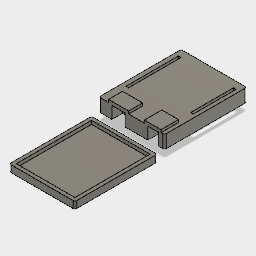
TentativeArduinoCase (Autodesk Fusion 360 design; units mm, degrees)
Autodesk Fusion 360 part; units mm, degrees
sketch "Sketch1" plane through (0, 0, 0) normal (0, 1, 0) x (1, 0, 0)
  line L0 (0, 0) -> (59.5312, 0)
  line L1 (59.5312, 0) -> (59.5312, 74.6125)
  line L2 (59.5312, 74.6125) -> (0, 74.6125)
  line L3 (0, 74.6125) -> (0, 0)
  dimension "d1" = 59.5312
  dimension "d2" = 74.6125
  constraint horizontal L0
  constraint vertical L1
  constraint horizontal L2
  constraint vertical L3
  constraint coincident L0.start L3.end
extrude "Extrude1" add sketch "Sketch1" against normal blind 6.35 makes body 1
sketch "Sketch2" plane through (0, 0, 0) normal (0, 1, 0) x (-1, 0, 0)
  line L0 (0, -74.6125) -> (0, 0)
  line L1 (0, 0) -> (-59.5312, 0)
  line L2 (-59.5312, 0) -> (-59.5312, -74.6125)
  line L3 (-59.5312, -74.6125) -> (0, -74.6125)
  line L4 (-56.3562, 0) -> (-41.275, 0)
  line L5 (-41.275, 0) -> (-56.3562, 0)
  line L6 (-41.275, 0) -> (-50.0063, 0)
  line L7 (-41.275, 0) -> (-56.3626, 0)
  line L8 (-56.3626, 0) -> (-56.3626, -15.875)
  line L9 (-56.3626, -15.875) -> (-41.275, -15.875)
  line L10 (-41.275, -15.875) -> (-41.275, 0)
  dimension "d6" = 15.0813
  dimension "d30" = 18.2563
  dimension "d31" = 15.875
  dimension "d93" = 15.0876
  constraint horizontal L6
  constraint horizontal L7
  constraint vertical L8
  constraint horizontal L9
  constraint vertical L10
  measures "d31" distance of L0.end
  measures "d93" distance of L8 L10
extrude "Extrude2" add sketch "Sketch2" along normal blind 14.2875 contours L1 L4 L5 L6 L7 L8 L9 L10 bodies 1
sketch "Sketch3" plane through (0, 0, 0) normal (0, 1, 0) x (-1, 0, 0)
  line L0 (-56.3626, 0) -> (-59.5312, 0)
  line L1 (-59.5312, 0) -> (-59.5312, -74.6125)
  line L2 (-59.5312, -74.6125) -> (0, -74.6125)
  line L3 (0, -74.6125) -> (0, 0)
  line L4 (0, 0) -> (-41.275, 0)
  line L5 (0, 0) -> (-26.9875, 0)
  line L6 (-26.9875, 0) -> (-8.7313, 0)
  line L7 (-8.7313, 0) -> (-20.6375, 0)
  line L8 (-8.7313, -12.7) -> (-8.7313, 0)
  line L9 (-56.3626, -15.875) -> (-56.3626, 0)
  line L10 (-41.275, 0) -> (-41.275, -15.875)
  line L11 (-41.275, -15.875) -> (-56.3626, -15.875)
  line L12 (-8.7313, -12.7) -> (-26.9875, -12.7)
  line L13 (-26.9875, -12.7) -> (-26.9875, 0)
  line L14 (-26.9875, 0) -> (-8.7313, 0)
  line L15 (-8.7313, 0) -> (-8.7313, -12.7)
  dimension "d10" = 26.9875
  dimension "d11" = 18.2563
  dimension "d12" = 12.7
  constraint coincident L3.end L4.start
  constraint coincident L5 L3.end
  constraint coincident L4 L3.end
  constraint horizontal L7
  constraint vertical L8
  constraint horizontal L12
  constraint vertical L13
  constraint horizontal L14
  constraint vertical L15
  measures "d12" distance of L3.end
extrude "Extrude3" add sketch "Sketch3" along normal blind 14.2875 contours L4 L5 L6 L7 L8 L12 L13 L14 L15 bodies 1
sketch "Sketch12" plane through (0, 0, 0) normal (0, 1, 0) x (-1, 0, 0)
  line L0 (-26.9875, -12.7) -> (-26.9875, 0)
  line L1 (-26.9875, 0) -> (-41.275, 0)
  line L2 (-41.275, 0) -> (-41.275, -15.875)
  line L3 (-41.275, -15.875) -> (-56.3626, -15.875)
  line L4 (-56.3626, -15.875) -> (-56.3626, 0)
  line L5 (-56.3626, 0) -> (-59.5312, 0)
  line L6 (-59.5312, 0) -> (-59.5312, -74.6125)
  line L7 (-59.5312, -74.6125) -> (0, -74.6125)
  line L8 (0, -74.6125) -> (0, 0)
  line L9 (0, 0) -> (-8.7313, 0)
  line L10 (-8.7313, 0) -> (-8.7313, -12.7)
  line L11 (-8.7313, -12.7) -> (-26.9875, -12.7)
  line L12 (0, 0) -> (-8.7313, 0)
  line L13 (-8.7313, 0) -> (-8.7313, -7.9375)
  line L14 (-8.7313, -7.9375) -> (0, -7.9375)
  line L15 (0, -7.9375) -> (0, 0)
  dimension "d57" = 7.9375
  constraint horizontal L12
  constraint vertical L13
  constraint horizontal L14
  constraint vertical L15
  constraint coincident L8.end L9.start
  measures "d57" distance of L8.end
extrude "Extrude10" add sketch "Sketch12" along normal blind 11.9062 bodies 1
sketch "Sketch13" plane through (0, 11.9062, 0) normal (0, 1, 0) x (-1, 0, 0)
  line L0 (-8.7313, -12.7) -> (-26.9875, -12.7)
  line L1 (-26.9875, -12.7) -> (-26.9875, 0)
  line L2 (0, 0) -> (-8.7313, 0)
  line L3 (-41.275, 0) -> (-41.275, -15.875)
  line L4 (-41.275, -15.875) -> (-56.3626, -15.875)
  line L5 (-56.3626, -15.875) -> (-56.3626, 0)
  line L6 (-56.3626, 0) -> (-59.5312, 0)
  line L7 (-59.5312, 0) -> (-59.5312, -74.6125)
  line L8 (-59.5312, -74.6125) -> (0, -74.6125)
  line L9 (0, -74.6125) -> (0, 0)
  line L10 (-8.7313, 0) -> (-8.7313, -12.7)
  line L11 (0, -74.6125) -> (-6.35, -74.6125)
  line L12 (-6.35, -74.6125) -> (-6.35, -20.6375)
  line L13 (-6.35, -20.6375) -> (0, -20.6375)
  line L14 (0, -20.6375) -> (0, -74.6125)
  line L15 (-59.5312, -74.6125) -> (-53.975, -74.6125)
  line L16 (-53.975, -74.6125) -> (-53.975, -29.3688)
  line L17 (-53.975, -29.3688) -> (-59.5312, -29.3688)
  line L18 (-59.5312, -29.3688) -> (-59.5312, -74.6125)
  line L19 (-26.9875, 0) -> (-41.275, 0)
  line L20 (0, -74.6125) -> (-3.9688, -74.6125)
  line L21 (-3.9688, -74.6125) -> (-3.9688, -20.6375)
  line L22 (-3.9688, -20.6375) -> (0, -20.6375)
  line L23 (0, -20.6375) -> (0, -74.6125)
  line L24 (0, -74.6125) -> (-6.35, -74.6125)
  line L25 (-6.35, -74.6125) -> (-6.35, -68.2625)
  line L26 (-6.35, -68.2625) -> (0, -68.2625)
  line L27 (0, -68.2625) -> (0, -74.6125)
  line L28 (-59.5312, -74.6125) -> (-56.3563, -74.6125)
  line L29 (-56.3563, -74.6125) -> (-56.3563, -29.3688)
  line L30 (-56.3563, -29.3688) -> (-59.5312, -29.3688)
  line L31 (-59.5312, -29.3688) -> (-59.5312, -74.6125)
  line L32 (-59.5312, -74.6125) -> (-53.975, -74.6125)
  line L33 (-53.975, -74.6125) -> (-53.975, -68.2625)
  line L34 (-53.975, -68.2625) -> (-59.5312, -68.2625)
  line L35 (-59.5312, -68.2625) -> (-59.5312, -74.6125)
  dimension "d60" = 53.975
  dimension "d61" = 6.35
  dimension "d62" = 45.2437
  dimension "d63" = 5.5563
  dimension "d94" = 53.975
  dimension "d95" = 3.9688
  dimension "d96" = 6.35
  dimension "d97" = 45.2437
  dimension "d98" = 3.175
  dimension "d99" = 6.35
  constraint horizontal L11
  constraint vertical L12
  constraint horizontal L13
  constraint vertical L14
  constraint coincident L2.start L9.end
  constraint horizontal L15
  constraint vertical L16
  constraint horizontal L17
  constraint vertical L18
  constraint horizontal L20
  constraint vertical L21
  constraint horizontal L22
  constraint vertical L23
  constraint horizontal L24
  constraint vertical L25
  constraint horizontal L26
  constraint vertical L27
  constraint horizontal L28
  constraint vertical L29
  constraint horizontal L30
  constraint vertical L31
  constraint coincident L12 L2.start
  constraint horizontal L32
  constraint vertical L33
  constraint horizontal L34
  constraint vertical L35
  constraint coincident L16 L2.start
  measures "d60" distance of L2.start
  measures "d94" distance of L2.start
extrude "Extrude11" cut sketch "Sketch13" against normal blind 11.9062 contours L12 L13 L21 L26 | L16 L17 L29 L34 bodies 1
sketch "Sketch14" plane through (0, 0, 0) normal (0, 0, 1) x (1, 0, 0)
  line L0 (0, 11.9062) -> (0, -6.35)
  line L1 (0, -6.35) -> (59.5312, -6.35)
  line L2 (59.5312, -6.35) -> (59.5312, 11.9063)
  line L3 (59.5312, 11.9062) -> (56.3626, 11.9062)
  line L4 (56.3626, 11.9062) -> (56.3626, 14.2875)
  line L5 (56.3626, 14.2875) -> (41.275, 14.2875)
  line L6 (41.275, 14.2875) -> (41.275, 11.9062)
  line L7 (41.275, 11.9062) -> (26.9875, 11.9062)
  line L8 (26.9875, 11.9062) -> (26.9875, 14.2875)
  line L9 (26.9875, 14.2875) -> (8.7313, 14.2875)
  line L10 (8.7313, 14.2875) -> (8.7313, 11.9062)
  line L11 (8.7313, 14.2875) -> (11.9063, 14.2875)
  line L12 (11.9063, 14.2875) -> (11.9063, 11.1125)
  line L13 (11.9063, 11.1125) -> (8.7313, 11.1125)
  line L14 (8.7313, 11.1125) -> (8.7313, 14.2875)
  line L15 (26.9875, 14.2875) -> (8.7313, 14.2875)
  line L16 (8.7313, 14.2875) -> (8.7313, 0)
  line L17 (8.7313, 0) -> (26.9875, 0)
  line L18 (26.9875, 0) -> (26.9875, 14.2875)
  line L19 (26.9875, 0) -> (23.8125, 0)
  line L20 (23.8125, 0) -> (23.8125, 3.175)
  line L21 (23.8125, 3.175) -> (26.9875, 3.175)
  line L22 (26.9875, 3.175) -> (26.9875, 0)
  line L23 (11.9063, 11.1125) -> (23.8125, 11.1125)
  line L24 (23.8125, 11.1125) -> (23.8125, 0)
  line L25 (23.8125, 0) -> (11.9063, 0)
  line L26 (11.9063, 0) -> (11.9063, 11.1125)
  line L27 (8.7313, 11.9062) -> (0, 11.9062)
  dimension "d66" = 3.175
  dimension "d67" = 3.175
  dimension "d68" = 3.175
  dimension "d69" = 3.175
  constraint horizontal L11
  constraint vertical L12
  constraint horizontal L13
  constraint vertical L14
  constraint perpendicular L15 L16
  constraint parallel L15 L17
  constraint parallel L16 L18
  constraint perpendicular L14 L15
  constraint horizontal L19
  constraint vertical L20
  constraint horizontal L21
  constraint vertical L22
  constraint horizontal L23
  constraint vertical L24
  constraint horizontal L25
  constraint vertical L26
  measures "d69" distance of origin
extrude "Extrude12" cut sketch "Sketch14" against normal blind 9.525 contours L17 L20 L23 L24 L25 L26 bodies 1
sketch "Sketch15" plane through (0, 0, 0) normal (0, 0, 1) x (1, 0, 0)
  line L0 (23.8125, 11.1125) -> (23.8125, 0)
  line L1 (23.8125, 0) -> (11.9063, 0)
  line L2 (11.9063, 0) -> (11.9063, 11.1125)
  line L3 (11.9063, 11.1125) -> (23.8125, 11.1125)
  line L4 (0, 11.9062) -> (0, -6.35)
  line L5 (0, -6.35) -> (59.5312, -6.35)
  line L6 (59.5312, -6.35) -> (59.5312, 11.9063)
  line L7 (59.5312, 11.9062) -> (56.3626, 11.9062)
  line L8 (56.3626, 11.9062) -> (56.3626, 14.2875)
  line L9 (56.3626, 14.2875) -> (41.275, 14.2875)
  line L10 (41.275, 14.2875) -> (41.275, 11.9062)
  line L11 (41.275, 11.9062) -> (26.9875, 11.9062)
  line L12 (26.9875, 11.9062) -> (26.9875, 14.2875)
  line L13 (26.9875, 14.2875) -> (8.7313, 14.2875)
  line L14 (8.7313, 14.2875) -> (8.7313, 11.9062)
  line L15 (41.275, 14.2875) -> (44.45, 14.2875)
  line L16 (44.45, 14.2875) -> (44.45, 11.1125)
  line L17 (44.45, 11.1125) -> (41.275, 11.1125)
  line L18 (41.275, 11.1125) -> (41.275, 14.2875)
  line L19 (56.3626, 14.2875) -> (53.1876, 14.2875)
  line L20 (53.1876, 14.2875) -> (53.1876, 11.1125)
  line L21 (53.1876, 11.1125) -> (56.3626, 11.1125)
  line L22 (56.3626, 11.1125) -> (56.3626, 14.2875)
  line L23 (44.45, 14.2875) -> (54.7687, 14.2875)
  line L24 (53.975, 0) -> (42.8625, 0)
  line L25 (44.45, 11.1125) -> (53.975, 11.1125)
  line L26 (53.975, 11.1125) -> (53.975, 0)
  line L27 (53.975, 0) -> (44.45, 0)
  line L28 (44.45, 0) -> (44.45, 11.1125)
  line L29 (8.7313, 11.9062) -> (0, 11.9062)
  dimension "d72" = 3.175
  dimension "d73" = 3.175
  dimension "d74" = 3.175
  dimension "d75" = 3.175
  constraint horizontal L15
  constraint vertical L16
  constraint horizontal L17
  constraint vertical L18
  constraint horizontal L19
  constraint vertical L20
  constraint horizontal L21
  constraint vertical L22
  constraint horizontal L23
  constraint horizontal L24
  constraint coincident origin
  constraint horizontal L25
  constraint vertical L26
  constraint horizontal L27
  constraint vertical L28
extrude "Extrude13" cut sketch "Sketch15" against normal blind 12.7 contours L21 L24 L25 L26 L27 L28 bodies 1
split "Split1" by plane through (0, 0, 0) normal (0, 1, 0) bodies 1 makes body 2 at (22.225, 11.9062, -39.4229)
move_body "MoveBody1" bodies 1 to x (1, 0, 0) y (0, 1, 0) z (0, 0, 1) at (0, 0, 81.28)
sketch "Sketch16" plane through (0, 0, 0) normal (0, 1, 0) x (-1, 0, 0)
  line L0 (0, 81.28) -> (-59.5312, 81.28)
  line L1 (-59.5312, 81.28) -> (-59.5312, 6.6675)
  line L2 (-59.5312, 6.6675) -> (0, 6.6675)
  line L3 (0, 6.6675) -> (0, 81.28)
  line L4 (0, 6.6675) -> (-3.175, 6.6675)
  line L5 (-3.175, 6.6675) -> (-3.175, 9.8425)
  line L6 (-3.175, 9.8425) -> (0, 9.8425)
  line L7 (0, 9.8425) -> (0, 6.6675)
  line L8 (-59.5312, 81.28) -> (-56.3563, 81.28)
  line L9 (-56.3563, 81.28) -> (-56.3563, 78.105)
  line L10 (-56.3563, 78.105) -> (-59.5312, 78.105)
  line L11 (-59.5312, 78.105) -> (-59.5312, 81.28)
  line L12 (-56.3563, 78.105) -> (-3.175, 78.105)
  line L13 (-3.175, 78.105) -> (-3.175, 9.8425)
  line L14 (-3.175, 9.8425) -> (-56.3563, 9.8425)
  line L15 (-56.3563, 9.8425) -> (-56.3563, 78.105)
  dimension "d78" = 3.175
  dimension "d79" = 3.175
  dimension "d80" = 3.175
  dimension "d81" = 3.175
  constraint horizontal L4
  constraint vertical L5
  constraint horizontal L6
  constraint vertical L7
  constraint horizontal L8
  constraint vertical L9
  constraint horizontal L10
  constraint vertical L11
  constraint horizontal L12
  constraint vertical L13
  constraint horizontal L14
  constraint vertical L15
  measures "d80" distance of origin
extrude "Extrude14" cut sketch "Sketch16" against normal blind 3.175 contours L12 L13 L14 L15 bodies 1
form "Form1" [no effect]
fillet "Fillet1" radius 1.5875 4 edges at (59.5312, -3.175, 81.28) (59.5312, -3.175, 6.6675) (0, -3.175, 81.28) (0, -3.175, 6.6675) on bodies 1
sketch "Sketch17" plane through (0, 0, 0) normal (0, -1, 0) x (1, 0, 0)
  line L0 (0, 0) -> (0, -74.6125)
  line L1 (0, -74.6125) -> (59.5312, -74.6125)
  line L2 (59.5312, -74.6125) -> (59.5312, 0)
  line L3 (11.9063, 0) -> (0, 0)
  line L4 (56.3563, -29.3688) -> (56.3563, -68.2625)
  line L5 (56.3563, -68.2625) -> (53.975, -68.2625)
  line L6 (53.975, -68.2625) -> (53.975, -29.3688)
  line L7 (53.975, -29.3688) -> (56.3563, -29.3688)
  line L8 (6.35, -68.2625) -> (3.9687, -68.2625)
  line L9 (3.9688, -68.2625) -> (3.9688, -20.6375)
  line L10 (3.9688, -20.6375) -> (6.35, -20.6375)
  line L11 (6.35, -20.6375) -> (6.35, -68.2625)
  line L12 (11.9063, -9.525) -> (11.9063, 0)
  line L13 (59.5312, 0) -> (53.975, 0)
  line L14 (53.975, 0) -> (53.975, -12.7)
  line L15 (53.975, -12.7) -> (44.45, -12.7)
  line L16 (44.45, -12.7) -> (44.45, 0)
  line L17 (23.8125, 0) -> (23.8125, -9.525)
  line L18 (23.8125, -9.525) -> (11.9063, -9.525)
  line L19 (53.975, -12.7) -> (53.975, -15.875)
  line L20 (59.5312, -15.875) -> (23.8188, -15.875)
  line L21 (23.8125, -9.525) -> (23.8125, -12.7)
  line L22 (23.8189, -15.875) -> (23.8125, -12.7)
  line L23 (23.8125, -12.7) -> (0, -12.7)
  line L24 (59.5312, -74.6125) -> (59.5312, -71.4375)
  line L25 (59.5312, -71.4375) -> (0, -71.4375)
  line L26 (53.975, -68.2625) -> (53.975, -71.4375)
  line L27 (6.35, -68.2625) -> (6.35, -71.4375)
  line L28 (56.3563, -68.2625) -> (56.3563, -71.4375)
  line L29 (3.9688, -68.2625) -> (3.9688, -71.4375)
  line L30 (56.3563, -29.3688) -> (56.3563, -15.875)
  line L31 (3.9688, -20.6375) -> (3.9687, -12.7)
  dimension "d100" = 3.175
  dimension "d101" = 4.7625
  dimension "d102" = 35.7188
  dimension "d103" = 35.7124
  dimension "d104" = 3.175
  dimension "d105" = 3.175
  constraint coincident L2
  constraint horizontal L20
  constraint coincident L20
  constraint coincident L0 L3.end
  constraint coincident L0.start L3.end
  constraint perpendicular L2 L25
  constraint coincident L25 L0.start
  constraint perpendicular L25 L26
  constraint perpendicular L25 L27
  constraint perpendicular L25 L28
  constraint perpendicular L25 L29
  constraint perpendicular L20 L30
  constraint coincident L23
  constraint perpendicular L23 L31
extrude "Extrude15" cut sketch "Sketch17" against normal blind 8.7313 contours L6 L7 L10 L11 L20 L22 L23 L25 L26 L27 L30 L31 | L8 L25 L27 L29 | L5 L25 L26 L28 bodies 2
fillet "Fillet2" radius 1.5875 4 edges at (59.5312, 5.9531, 0) (59.5312, 5.9531, -74.6125) (0, 5.9531, -74.6125) (0, 5.9531, 0) on bodies 2
equation "d1 = ( ( 67 / 32 ) * 1 in ) + 0.25 in"
equation "d2 = ( ( 86 / 32 ) * 1 in ) + 0.25 in"
equation "d3 = ( -1 / 4 ) * 1 in"
equation "d6 = ( ( 11 / 32 ) * 1 in ) + ( 1 / 4 ) * 1 in"
equation "d8 = ( 18 / 32 ) * 1 in"
equation "d10 = ( ( 26 / 32 ) * 1 in ) + ( 1 / 4 ) * 1 in"
equation "d11 = ( ( 15 / 32 ) * 1 in ) + ( 1 / 4 ) * 1 in"
equation "d12 = ( ( 12 / 32 ) * 1 in ) + ( 1 / 8 ) * 1 in"
equation "d13 = ( 18 / 32 ) * 1 in"
equation "d30 = ( ( 15 / 32 ) * 1 in ) + ( 1 / 4 ) * 1 in"
equation "d31 = ( 1 / 2 ) * 1 in + ( 1 / 8 ) * 1 in"
equation "d57 = ( 5 / 16 ) * 1 in"
equation "d58 = ( 11 / 32 ) * 1 in + ( 1 / 8 ) * 1 in"
equation "d61 = ( 1 / 4 ) * 1 in"
equation "d62 = ( 21 / 32 ) * 1 in + 1 in + 0.125 in"
equation "d63 = ( 0.25 ) * 1 in - ( 1 / 32 ) * 1 in"
equation "d64 = ( -15 / 32 ) * 1 in"
equation "d66 = ( 1 / 8 ) * 1 in"
equation "d67 = ( 1 / 8 ) * 1 in"
equation "d68 = ( 1 / 8 ) * 1 in"
equation "d69 = ( 1 / 8 ) * 1 in"
equation "d70 = ( -12 / 32 ) * 1 in"
equation "d72 = ( 1 / 8 ) * 1 in"
equation "d73 = ( 1 / 8 ) * 1 in"
equation "d74 = ( 1 / 8 ) * 1 in"
equation "d75 = ( 1 / 8 ) * 1 in"
equation "d76 = ( -16 / 32 ) * 1 in"
equation "d78 = ( 1 / 8 ) * 1 in"
equation "d79 = ( 1 / 8 ) * 1 in"
equation "d80 = ( 1 / 8 ) * 1 in"
equation "d81 = ( 1 / 8 ) * 1 in"
equation "d82 = ( -1 / 8 ) * 1 in"
equation "d84 = ( 1 / 16 ) * 1 in"
equation "d94 = 2 in + ( 1 / 8 ) * 1 in"
equation "d95 = ( 1 / 8 ) * 1 in + ( 1 / 32 ) * 1 in"
equation "d96 = ( 1 / 4 ) * 1 in"
equation "d97 = ( 21 / 32 ) * 1 in + 1 in + 0.125 in"
equation "d99 = ( 1 / 4 ) * 1 in"
equation "d100 = ( 1 / 8 ) * 1 in"
equation "d104 = ( 1 / 8 ) * 1 in"
equation "d105 = ( 1 / 8 ) * 1 in"
equation "d106 = ( -11 / 32 ) * 1 in"
equation "d108 = ( 1 / 16 ) * 1 in"
